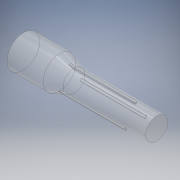
# Autodesk Inventor part: LED Pipe
Saved by Autodesk Inventor 2017 (Build 210142000, 142)
## iProperties
Created: 2018-07-19
Part Number: LED Pipe
Material: Polycarbonate, Clear
Document SubType Name: Modeling
Designer: intelsath
Density: 1.2 g/cm^3
Appearance: Polycarbonate - Clear
Author: intelsath
Autodesk Inventor part; units mm, degrees
ref_plane "YZ Plane" through (0, 0, 0) normal (1, 0, 0) x (0, 1, 0)
ref_plane "XZ Plane" through (0, 0, 0) normal (0, 1, 0) x (-1, 0, 0)
ref_plane "XY Plane" through (0, 0, 0) normal (0, 0, 1) x (1, 0, 0)
sketch "Sketch1" plane through (0, 0, 0) normal (0, 0, 1) x (1, 0, 0)
  line L0 (0, 0) -> (6.02, 0)
  line L1 (6.02, 0) -> (6.02, 0.495)
  line L2 (6.02, 0.495) -> (2.29, 0.495)
  line L3 (2.29, 0.495) -> (1.63, 0.735)
  line L4 (1.63, 0.735) -> (0, 0.735)
  line L5 (0, 0.735) -> (0, 0)
  dimension "d1" = 0.495
  dimension "d19" = 1.63
  dimension "d20" = 0.735
  dimension "d21" = 6.02
  dimension "d22" = 3.73
  constraints: 12 end point, 3 perpendicular, 2 horizontal
  measures "d1" distance of L0.end L1.end
  measures "d19" distance of L3.end L4.end
  measures "d20" distance of L4.end L0.start
  measures "d21" distance between parallel lines of L5 L1
  measures "d22" distance of L1.end L2.end
revolve "Revolution1" add sketch "Sketch1" angle 360 about axis through (0, 0, 0) along (1, 0, 0)
sketch "Sketch2" plane through (0, 0, 0) normal (-1, 0, 0) x (0, 0, 1)
  line L0 (0.36, 0.05) -> (0.56, 0.05)
  line L1 (0.56, 0.05) -> (0.56, -0.05)
  line L2 (0.56, -0.05) -> (0.36, -0.05)
  line L3 (0.36, -0.05) -> (0.36, 0.05)
  line L4 (-0.2233, 0.2868) -> (-0.3233, 0.46)
  line L5 (-0.3233, 0.46) -> (-0.2367, 0.51)
  line L6 (-0.2367, 0.51) -> (-0.1367, 0.3368)
  line L7 (-0.1367, 0.3368) -> (-0.2233, 0.2868)
  line L8 (-0.1367, -0.3368) -> (-0.2367, -0.51)
  line L9 (-0.2367, -0.51) -> (-0.3233, -0.46)
  line L10 (-0.3233, -0.46) -> (-0.2233, -0.2868)
  line L11 (-0.2233, -0.2868) -> (-0.1367, -0.3368)
  circle A0 centre (0, 0) radius 0.495 construction
  point P0 (0.36, 0)
  dimension "d9" = 360
  dimension "d23" = 0.56
  dimension "d24" = 0.1
  dimension "d25" = 0.2
  constraints: 24 end point, 2 parallel, 1 coincident, 1 horizontal, 1 horizontal alignment, 1 midpoint, 1 perpendicular, 25 other
  measures "d23" distance from line of point (0, 0) L5
  measures "d24" distance of L0.end L1.end
  measures "d25" distance of L0.start L0.end
extrude "Extrusion1" add sketch "Sketch2" against normal blind 5.08
body "Solid1"
